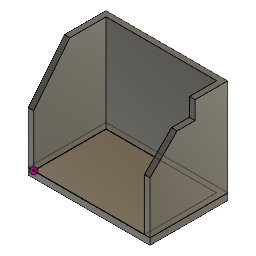
battery holder v1 (Autodesk Fusion 360 design; units mm, degrees)
Autodesk Fusion 360 part; units mm, degrees
sketch "Sketch1" plane through (0, 0, 0) normal (0, 0, 1) x (1, 0, 0)
  line L0 (0, 0) -> (49, 0)
  line L1 (49, 0) -> (49, 32)
  line L2 (49, 32) -> (0, 32)
  line L3 (0, 32) -> (0, 0)
  line L4 (0, 0) -> (-2.5, 0)
  line L5 (-2.5, 0) -> (51.5, 0)
  line L6 (51.5, 0) -> (51.5, 34.5)
  line L7 (51.5, 34.5) -> (-2.5, 34.5)
  line L8 (-2.5, 34.5) -> (-2.5, 0)
  dimension "d1" = 49
  dimension "d2" = 32
  dimension "d3" = 2.5
  dimension "d4" = 34.5
  dimension "d5" = 54
  constraint horizontal L0
  constraint vertical L1
  constraint horizontal L2
  constraint vertical L3
  constraint coincident L0.start L3.end
  constraint perpendicular L3 L4
  constraint horizontal L5
  constraint vertical L6
  constraint horizontal L7
  constraint vertical L8
  measures "d1" distance of L0.start L0.end
  measures "d2" distance of L0.start L2.end
  measures "d3" distance of L0.start L4.end
  measures "d4" distance of L4.end L7.end
  measures "d5" distance of L4.end L5.end
extrude "Extrude1" add sketch "Sketch1" against normal blind 3
sketch "Sketch2" plane through (0, 0, 0) normal (0, 1, 0) x (1, 0, 0)
extrude "Extrude2" add sketch "Sketch1" along normal blind 43 contours L1 L2 L3 L4 L5 L6 L7 L8
sketch "Sketch3" plane through (51.5, 0, 0) normal (1, 0, 0) x (0, 1, 0)
  line L0 (0, 43) -> (0, -3)
  line L1 (0, -3) -> (34.5, -3)
  line L2 (34.5, -3) -> (34.5, 43)
  line L3 (34.5, 43) -> (0, 43)
  line L4 (34.5, 43) -> (32, 43)
  line L5 (32, 43) -> (0, 43)
  line L6 (0, 43) -> (16, 43)
  line L7 (16, 43) -> (12, 43)
  line L8 (12, 43) -> (12, 35)
  line L9 (12, 35) -> (16, 35)
  line L10 (16, 35) -> (16, 43)
  line L11 (16, 43) -> (20, 43)
  line L12 (20, 43) -> (20, 35)
  line L13 (20, 35) -> (16, 35)
  line L14 (16, 35) -> (16, 43)
  point P0 (32, 43)
  point P1 (32, 43)
  dimension "d10" = 4
  dimension "d11" = 8
  dimension "d12" = 8
  constraint coincident L2.end L3.start
  constraint coincident P1 P0
  constraint coincident L0.start L3.end
  constraint midpoint L5 L6.end
  constraint horizontal L7
  constraint vertical L8
  constraint horizontal L9
  constraint vertical L10
  constraint horizontal L11
  constraint vertical L12
  constraint horizontal L13
  constraint vertical L14
  measures "d10" distance of L6.end L7.end
  measures "d11" distance of L6.end L9.end
  measures "d12" distance of L6.end L9.end
extrude "Extrude3" cut sketch "Sketch3" against normal blind 10 contours L3 L5 L6 L7 L8 L9 L10 L14 | L3 L5 L10 L11 L12 L13 L14
sketch "Sketch4" plane through (51.5, 0, 0) normal (1, 0, 0) x (0, 1, 0)
  line L0 (20, 43) -> (20, 35)
  line L1 (20, 35) -> (12, 35)
  line L2 (12, 35) -> (12, 43)
  line L3 (12, 43) -> (0, 43)
  line L4 (0, 43) -> (0, -3)
  line L5 (0, -3) -> (34.5, -3)
  line L6 (34.5, -3) -> (34.5, 43)
  line L7 (34.5, 43) -> (20, 43)
  line L8 (0, 43) -> (0, 23)
  line L9 (0, 23) -> (12, 35)
  dimension "d15" = 20
  constraint coincident L3.end L4.start
  constraint perpendicular L3 L8
  constraint coincident L1.end L2.start
  measures "d15" distance of L3.end L8.end
extrude "Extrude4" cut sketch "Sketch4" against normal blind 5 contours L2 L3 L4 L8 L9
sketch "Sketch5" plane through (-2.5, 0, 0) normal (-1, 0, 0) x (0, -1, 0)
  line L0 (-34.5, 43) -> (-34.5, -3)
  line L1 (-34.5, -3) -> (0, -3)
  line L2 (0, -3) -> (0, 43)
  line L3 (0, 43) -> (-34.5, 43)
  line L4 (0, 43) -> (-16, 43)
  line L5 (0, 43) -> (0, 23)
  line L6 (-16, 43) -> (0, 23)
  dimension "d18" = 16
  dimension "d19" = 20
  constraint coincident L2.end L3.start
  constraint perpendicular L2 L4
  constraint perpendicular L3 L5
  measures "d18" distance of L2.end L4.end
  measures "d19" distance of L2.end L5.end
extrude "Extrude5" cut sketch "Sketch5" against normal blind 10 contours L2 L3 L4 L5 L6
